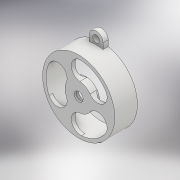
# Autodesk Inventor part: pitchThings
Saved by Autodesk Inventor 2018.2 (Build 222227000, 227)
## iProperties
Created: 2018-03-30
Part Number: pitchThings
Material: ABS Plastic
Document SubType Name: Modeling
Designer: Muchen He
Density: 1.06 g/cm^3
Appearance: Smooth - White
Author: Muchen He
Autodesk Inventor part; units mm, degrees
ref_plane "YZ Plane" through (0, 0, 0) normal (1, 0, 0) x (0, 1, 0)
ref_plane "XZ Plane" through (0, 0, 0) normal (0, 1, 0) x (-1, 0, 0)
ref_plane "XY Plane" through (0, 0, 0) normal (0, 0, 1) x (1, 0, 0)
sketch "Sketch1" plane through (0, 0, 0) normal (0, 1, 0) x (-1, 0, 0)
  circle A0 centre (0, 0) radius 19
  circle A1 centre (0, 0) radius 21
  circle A2 centre (0, 0) radius 4.9
  circle A3 centre (0, 0) radius 2.5875
  arc A4 (12.235155, -5.705347) -> (12.235155, 5.705347) centre (0, 0) ccw construction
  arc A5 (17.219848, -8.029747) -> (17.219848, 8.029747) centre (0, 0) ccw
  arc A6 (7.250462, -3.380946) -> (7.250462, 3.380946) centre (0, 0) ccw
  arc A7 (7.250462, -3.380946) -> (17.219848, -8.029747) centre (12.235155, -5.705347) ccw
  arc A8 (17.219848, 8.029747) -> (7.250462, 3.380946) centre (12.235155, 5.705347) ccw
  line L0 (12.235155, 5.705347) -> (0, 0) construction
  line L1 (0, 0) -> (12.235155, -5.705347) construction
  circle A9 centre (0, 0) radius 8
  point P0 (13.5, 0)
  dimension "d0" = 42
  dimension "d1" = 2
  dimension "d2" = 9.8
  dimension "d3" = 5.175
  dimension "d4" = 50
  dimension "d7" = 8
  constraints: 11 point on circle, 9 centre point, 5 coincident, 4 end point, 4 tangent, 2 concentric, 1 horizontal alignment, 3 other
  measures "d0" diameter of A1
  measures "d1" radial gap between concentric circles of A1 A0
  measures "d2" diameter of A2
  measures "d3" diameter of A3
  measures "d4" angle of L0 L1
  measures "d7" radius of A6
extrude "Extrusion1" add sketch "Sketch1" against normal blind 1.15 contours A0 A7 A6 A8 | A8 A9 A7 A0 | A6 A9 | A1
sketch "Sketch3" plane through (0, -1.15, 0) normal (0, -1, 0) x (1, 0, 0)
  circle A0 centre (0, 0) radius 4.9 projected
  circle A1 centre (0, 0) radius 21 projected
  circle A2 centre (0, 0) radius 2.5875 projected
extrude "Extrusion5" add sketch "Sketch3" along normal blind 1 contours A0 | A1
extrude "Extrusion6" add sketch "Sketch1" along normal blind 2 contours A6 A9
extrude "Extrusion2" cut sketch "Sketch1" against normal up to next contours A0 A7 A6 A8
pattern_circular "Circular Pattern1" count 3 over 360 about axis through (0, -10, 0) along (0, 1, 0) of "Extrusion2"
extrude "Extrusion3" add sketch "Sketch1" along normal blind 11 contours A1
sketch "Sketch2" plane through (0, 11, 0) normal (0, 1, 0) x (1, 0, 0)
  circle A0 centre (0, -24) radius 2
  circle A1 centre (0, 24) radius 2
  line L0 (0, -24) -> (0, 24) construction
  line L1 (-4, -20.615528) -> (-4, -24)
  arc A2 (-4, -24) -> (4, -24) centre (0, -24) ccw
  line L2 (4, -24) -> (4, -20.615528)
  line L3 (-4, 20.615528) -> (-4, 24)
  arc A3 (4, 24) -> (-4, 24) centre (0, 24) ccw
  line L4 (4, 24) -> (4, 20.615528)
  circle A4 centre (0, 0) radius 21
  dimension "d15" = 48
  dimension "d16" = 4
  dimension "d17" = 4
  constraints: 10 end point, 4 centre point, 4 point on circle, 4 tangent, 3 vertical, 2 concentric, 2 equal radius, 2 midpoint, 1 coincident, 1 parallel, 1 vertical alignment
  measures "d15" distance of L0.start L0.end
  measures "d16" diameter of A1
  measures "d17" radius of A3
extrude "Extrusion4" add sketch "Sketch2" against normal blind 3 contours A4 L2 A2 L1 | L3 A3 L4 A4
fillet "Fillet1" radius 2 3 edges at (-4, 0, -6.9282) (8, 0, 0) (-4, 0, 6.9282)
body "Solid1"
